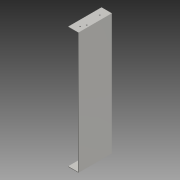
# Autodesk Inventor part: bewegliche achse horizontal
Saved by Autodesk Inventor 2013 (Build 170138000, 138)
## iProperties
Created: 2012-10-21
Part Number: bewegliche achse horizontal
Material: Stahl
Document SubType Name: Modeling
Designer: fivef
Density: 7.85 g/cm^3
Mass: 678.536 g
Surface Area: 1170.39 cm^2
Volume: 86.4377 cm^3
Author: fivef
Autodesk Inventor part; units mm, degrees
ref_plane "YZ Plane" through (0, 0, 0) normal (1, 0, 0) x (0, 1, 0)
ref_plane "XZ Plane" through (0, 0, 0) normal (0, 1, 0) x (-1, 0, 0)
ref_plane "XY Plane" through (0, 0, 0) normal (0, 0, 1) x (1, 0, 0)
sketch "Skizze1" plane through (0, 0, 0) normal (0, 0, 1) x (1, 0, 0)
  line L0 (-17, -55) -> (17, -55)
  line L1 (17, -55) -> (17, 55)
  line L2 (17, 55) -> (-17, 55)
  line L3 (-17, 55) -> (-17, -55)
  line L4 (-17, 55) -> (17, -55) construction
  line L5 (-17, -55) -> (17, 55) construction
  point P0 (0, 0)
  point P1 (0, 0)
  dimension "d0" = 34
  dimension "d2" = 110
  constraints: 12 end point, 2 parallel, 1 coincident, 1 horizontal, 1 midpoint, 1 perpendicular
  measures "d0" distance of L0.end L0.start
  measures "d2" distance of L0.end L1.end
extrude "Extrusion1" add sketch "Skizze1" along normal mid plane 400
sketch "Skizze2" plane through (0, 0, 200) normal (0, 0, 1) x (1, 0, 0)
  line L0 (-17, -55) -> (17, -55) projected
  line L1 (17, -55) -> (17, 55) projected
  line L2 (17, 55) -> (-17, 55) projected
  point P0 (0, 0)
  point P1 (2, 30)
  point P2 (9, -20)
  point P3 (2, -35)
  dimension "d5" = 25
  dimension "d6" = 15
  dimension "d30" = 50
  dimension "d31" = 8
  dimension "d32" = 7
  dimension "d33" = 35
  dimension "d40" = 20
  dimension "d41" = 15
  measures "d5" distance from line of L2 point (2, 30)
  measures "d6" distance from line of L1 point (2, 30)
  measures "d30" vertical distance of point (2, 30) point (9, -20)
  measures "d31" distance from line of point (9, -20) L1
  measures "d32" horizontal distance of point (2, 30) point (9, -20)
  measures "d33" distance from line of L0 point (9, -20)
  measures "d40" distance from line of point (2, -35) L0
  measures "d41" distance from line of L1 point (2, -35)
hole "Bohrung1" at (2, 30, 200) at (9, -20, 200) at (2, -35, 200) direction (0, 0, -1) diameter 4 end through all
sketch "Skizze4" plane through (-17, -55, 200) normal (-1, 0, 0) x (0, 0, 1)
  line L0 (0, 0) -> (-400, 0) projected
  line L1 (0, 110) -> (0, 0) projected
  line L2 (-400, 110) -> (0, 110) projected
  line L3 (-400, 0) -> (-400, 110) projected
  line L4 (-398.5, 108.5) -> (-1.5, 108.5)
  line L5 (-1.5, 108.5) -> (-1.5, 0)
  line L6 (-1.5, 0) -> (-398.5, 0)
  line L7 (-398.5, 0) -> (-398.5, 108.5)
  point P0 (-200, 55)
  dimension "d34" = 1.5
  dimension "d35" = 0
  dimension "d36" = 1.5
  dimension "d37" = 1.5
  constraints: 8 end point, 2 parallel, 1 horizontal, 1 perpendicular
  measures "d34" distance between parallel lines of L2 L4
  measures "d35" distance between parallel lines of L0 L6
  measures "d36" distance between parallel lines of L1 L5
  measures "d37" distance between parallel lines of L3 L7
extrude "Extrusion2" cut sketch "Skizze4" against normal blind 32.5 contours L0 L7 L4 L5
sketch "Skizze5" plane through (-17, 55, 200) normal (0, 1, 0) x (1, 0, 0)
  line L0 (34, 0) -> (0, 0) projected
  line L1 (34, 400) -> (34, 0) projected
  line L2 (0, 400) -> (34, 400) projected
  line L3 (0, 398.5) -> (16, 398.5)
  line L4 (16, 398.5) -> (16, 1.5)
  line L5 (16, 1.5) -> (0, 1.5)
  line L6 (0, 1.5) -> (0, 398.5)
  point P0 (17, 200)
  dimension "d42" = 1.5
  dimension "d43" = 1.5
  dimension "d44" = 18
  constraints: 8 end point, 2 parallel, 1 horizontal, 1 perpendicular
  measures "d42" distance between parallel lines of L2 L3
  measures "d43" distance between parallel lines of L0 L5
  measures "d44" distance between parallel lines of L1 L4
extrude "Extrusion3" cut sketch "Skizze5" against normal blind 32.5
